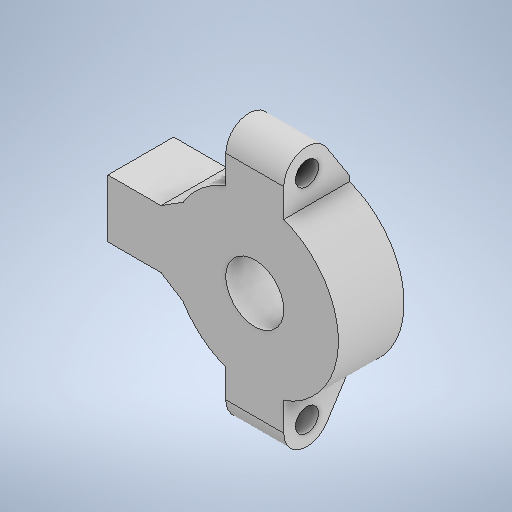
# Autodesk Inventor part: NewCameraHolder
Saved by Autodesk Inventor 2025.1 (Build 291241000, 241)
## iProperties
Created: 2026-05-18
Part Number: NewCameraHolder
Material: Generic
Document SubType Name: Modeling
Designer: User
Density: 1 g/cm^3
Appearance: Default
Author: User
## iProperties of the stored document NewCameraHolder_3DPrint.ipt
Created: 2026-05-18
Part Number: NewCameraHolder_3DPrint
Material: Generic
Document SubType Name: Modeling
Designer: User
Density: 1 g/cm^3
Appearance: Default
Author: User
Autodesk Inventor part; units mm, degrees
ref_plane "YZ Plane" through (0, 0, 0) normal (1, 0, 0) x (0, 1, 0)
ref_plane "XZ Plane" through (0, 0, 0) normal (0, 1, 0) x (-1, 0, 0)
ref_plane "XY Plane" through (0, 0, 0) normal (0, 0, 1) x (1, 0, 0)
sketch "Sketch1" plane through (0, 0, 0) normal (0, 0, 1) x (1, 0, 0)
  circle A0 centre (0, 0) radius 3.75 projected
  line L0 (10.8, -10.8193) -> (10.8234, 10.804) projected
  line L1 (-10.8, 10.8274) -> (-10.8234, -10.7959) projected
  arc A1 (-10.1405, -3.75) -> (-10.1405, 3.75) centre (0, 0) ccw
  line L2 (0, 3.75) -> (-19, 3.75)
  line L3 (0, 3.75) -> (19, 3.75) construction
  line L4 (-19, 3.75) -> (-19, -3.75)
  line L5 (-19, -3.75) -> (0, -3.75)
  point P0 (0, 0)
  dimension "d0" = 19
  dimension "d1" = 180
  constraints: 8 end point, 4 point on circle, 2 horizontal, 2 point on line, 2 tangent, 1 centre point, 1 coincident, 1 collinear, 1 perpendicular
  measures "d0" distance of L2.start L2.end
  measures "d1" angle of L2 L3
extrude "Extrusion1" add sketch "Sketch1" along normal blind 8.5 contours A0 L2 A1 L5 | A0 L5 L1 L2 | L1 L5 L4 L2
sketch "Sketch2" plane through (0, 0, 8.5) normal (0, 0, 1) x (1, 0, 0)
  arc A0 (-10.1405, -3.75) -> (-10.1405, 3.75) centre (0, 0) ccw projected
  circle A1 centre (0, 0) radius 3.75 projected
  circle A2 centre (0, 0) radius 3.75 projected
  line L0 (3.75, 0) -> (3.75, 10.8117)
  line L1 (0, 10.8117) -> (3.75, 10.8117)
  line L2 (-3.75, 0) -> (-3.75, 10.8117)
  line L3 (-3.75, 10.8117) -> (3.75, 10.8117)
  line L4 (0, -10.8117) -> (-3.75, -10.8117)
  line L5 (-3.75, -10.8117) -> (-3.75, 0)
  line L6 (3.75, 0) -> (3.75, -10.8117)
  line L7 (3.75, -10.8117) -> (-3.75, -10.8117)
  point P0 (0, 0)
  point P1 (-3.75, 10.1405)
  point P2 (3.75, 10.1405)
  point P3 (3.75, -10.1405)
  point P4 (-3.75, -10.1405)
  constraints: 16 end point, 9 tangent, 4 perpendicular, 4 point on circle, 1 collinear, 1 horizontal, 1 parallel, 1 point on line, 1 vertical
extrude "Extrusion2" add sketch "Sketch2" against normal up to surface (8.5 mm away) contours A0 L4 L5 | A0 L6 L7 | L2 L3 A0 | A0 L1 L0
sketch "Sketch3" plane through (-3.75, -10.8117, 8.5) normal (-1, 0, 0) x (0, 0, 1)
  line L0 (0, 0) -> (-8.5, 0) projected
  line L1 (0, 21.6234) -> (-8.5, 21.6234) projected
  line L2 (0, 0) -> (0, 0.6712) projected
  line L3 (0, 0) -> (-6, 0)
  line L4 (0, 0) -> (-8.5, 0) projected
  line L5 (0, 0) -> (-3, 0)
  line L6 (-3, 0) -> (-3, -6)
  line L7 (-3, 0) -> (3, 0) construction
  circle A0 centre (-3, -3) radius 1.5
  line L8 (0, 21.6234) -> (-3, 21.6234)
  line L9 (-3, 21.6234) -> (-3, 27.6234)
  circle A1 centre (-3, 24.6234) radius 1.5
  circle A2 centre (-3, 24.6234) radius 3
  circle A3 centre (-3, -3) radius 3
  line L10 (0, 0) -> (0, -3)
  line L11 (-8.5, 0) -> (-5.5223, -4.6242)
  line L12 (0, 21.6234) -> (0, 24.6234)
  line L13 (0, 21.6234) -> (-8.5, 21.6234) projected
  line L14 (-8.5, 21.6234) -> (-5.5223, 26.2476)
  point P0 (-8.5, 10.8117)
  dimension "d6" = 6
  dimension "d7" = 3
  dimension "d8" = 6
  dimension "d9" = 90
  dimension "d10" = 3
  dimension "d11" = 3
  dimension "d12" = 6
  dimension "d13" = 3
  constraints: 20 end point, 6 point on circle, 4 centre point, 4 tangent, 3 point on line, 2 coincident, 2 midpoint, 2 perpendicular, 1 horizontal, 1 vertical
  measures "d6" distance of L0.start L3.end
  measures "d7" distance of L0.start L5.end
  measures "d8" distance of L5.end L6.end
  measures "d9" angle of L6 L7
  measures "d10" diameter of A0
  measures "d11" distance of L1.start L8.end
  measures "d12" distance of L8.end L9.end
  measures "d13" diameter of A1
extrude "Extrusion3" add sketch "Sketch3" against normal up to surface (7.5 mm away) contours L10 A3 L0 | A3 L11 L0 | A3 L6 A0 | L6 A0 A3 | L1 A2 L12 | A2 L9 A1 | L1 L14 A2 | L9 A1 A2
chamfer "Chamfer1" distance 2 angle 45 2 edges at (-10.1405, -3.75, 4.25) (-10.1405, 3.75, 4.25)
body "Solid1"
